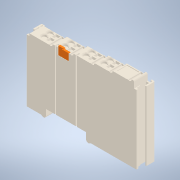
# Autodesk Inventor part: 750-530
Saved by Autodesk Inventor 2021 (Build 250183000, 183)
## iProperties
Created: 2026-07-30
Part Number: 750-530
Material: Generic
Catalog Web Link: www.3dfindit.com
Description: 750-530-8-channel digital output module 24 VDC 0.5 A high-side switching short-circuit protected
Vendor: WAGO
Document SubType Name: Modeling
Designer: psAdmin
Manufacturer: WAGO
Mass: 49.754 g
Surface Area: 192.522 cm^2
Volume: 65.9871 cm^3
Density: 1 g/cm^3
Appearance: PSOLRGB-222-214-201
Category: PARTsolutions
Company: WAGO
Title: 750-530
Author: Cadenas PARTsolutions
Comments: 8-channel digital output module 24 VDC 0.5 A high-side switching short-circuit protected
PSOL_IDENT_0: {$CADENAS_DATA/23d-libs/wago/pg15/serie750/0750-0530_0999-0962.prj},157 {VTYP=3D},{NB=750-530},{LINA=
PSOL_IDENT_1: 750-530},{NN=750-530},{DATE=29.04.2026 11:59:10},{GEOMDATE=22.04.2022 08:42:40},{VERSION=},{LINEID=1
PSOL_IDENT_2: 710},{WBVAR=},{WBNUMERIC=}  {NB=750-530},{LINA=750-530},{KT=DUMMY},{BESTNR=750-530},{INFODE=Info DE}
PSOL_IDENT_3: ,{INFOEN=Info EN},{QUERSCHNITT1=0.08 - 2.5},{QUERSCHNITT2=28 - 14},{ABISOLIERLAENGE=8 - 9},{HOEHE=64
PSOL_IDENT_4: .00},{BREITE=12.00},{TIEFE=100.00},{FARBE=lichtgrau},{GEWICHT=49.754},{BEMERKUNGEN=24V DC 0,5 A},{RG
PSOL_IDENT_5: B=0.87,0.84,0.79,0},{ECLASS71=27-24-26-04},{LINKDE=http://www.wago.com/de/p/750-530},{LINKEN=http://
PSOL_IDENT_6: www.wago.com/global/p/750-530},{FILENAME=750-530}
NB: 750-530
NN: 750-530
NT: 8-channel digital output module 24 VDC 0.5 A high-side switching short-circuit protected
NBSYN: $BESTNR.
LINA: 750-530
CATALOG: WAGO
OFFICIAL_STANDARD_NUMBERS: NO
BESTNR: 750-530
INFODE: Info DE
INFOEN: Info EN
QUERSCHNITT1: 0.08 - 2.5
QUERSCHNITT2: 28 - 14
ABISOLIERLAENGE: 8 - 9
HOEHE: 64
BREITE: 12
TIEFE: 100
FARBE: lichtgrau
GEWICHT: 49.754
BEMERKUNGEN: 24V DC 0,5 A
ECLASS71: 27-24-26-04
SUPPLIER: WAGO
ARTICLENO: 750-530
BOMINFO: 750-530
CREATOR: CADENAS GmbH
Autodesk Inventor part; units mm, degrees
ref_plane "YZ Plane" through (0, 0, 0) normal (1, 0, 0) x (0, 1, 0)
ref_plane "XZ Plane" through (0, 0, 0) normal (0, 1, 0) x (-1, 0, 0)
ref_plane "XY Plane" through (0, 0, 0) normal (0, 0, 1) x (1, 0, 0)
sketch "Skizze_1" plane through (0, 0, 0) normal (0, 0, 1) x (1, 0, 0)
  line L0 (-32.4, 49.7072) -> (-32.4, -6.4)
  line L1 (-32.4, -6.4) -> (-21.9679, -6.4)
  line L2 (-21.9679, -6.4) -> (-20.7, -7.1321)
  arc A0 (-20.7, -7.1321) -> (-17.7, -5.4) centre (-19.7, -5.4) ccw
  line L3 (-17.7, -5.4) -> (-17.7, 0)
  line L4 (-17.7, 0) -> (17.7, 0)
  line L5 (17.7, 0) -> (17.7, -5.4)
  arc A1 (17.7, -5.4) -> (20.7, -7.1321) centre (19.7, -5.4) ccw
  line L6 (20.7, -7.1321) -> (21.9679, -6.4)
  line L7 (21.9679, -6.4) -> (60, -6.4)
  line L8 (60, -6.4) -> (60, 59.4)
  arc A2 (60, 59.4) -> (59, 60.4) centre (59, 59.4) ccw
  line L9 (59, 60.4) -> (58.8171, 60.4)
  arc A3 (58.8171, 60.4) -> (58.5293, 60.2779) centre (58.8171, 60) ccw
  line L10 (58.5293, 60.2779) -> (58.4531, 60.1989)
  arc A4 (58.4531, 60.1989) -> (58.6439, 59.6405) centre (58.6915, 59.9686) ccw
  arc A5 (59.0357, 58.9584) -> (58.6439, 59.6405) centre (58.5721, 59.1457) ccw
  line L11 (59.0357, 58.9584) -> (58.9581, 58.7664)
  line L12 (58.9581, 58.7664) -> (54.8948, 57.0416)
  line L13 (54.8948, 57.0416) -> (54.7028, 57.1192)
  arc A6 (54.4842, 57.8749) -> (54.7028, 57.1192) centre (54.8901, 57.5828) ccw
  arc A7 (54.4842, 57.8749) -> (54.2152, 58.4) centre (54.2152, 58.0685) ccw
  line L14 (54.2152, 58.4) -> (41.9117, 58.4)
  line L15 (41.9117, 58.4) -> (41.8025, 58.3537)
  line L16 (41.8025, 58.3537) -> (41.6531, 58.1989)
  arc A8 (41.6531, 58.1989) -> (41.8439, 57.6405) centre (41.8915, 57.9686) ccw
  arc A9 (42.2357, 56.9584) -> (41.8439, 57.6405) centre (41.7721, 57.1457) ccw
  line L17 (42.2357, 56.9584) -> (42.1581, 56.7664)
  line L18 (42.1581, 56.7664) -> (38.0948, 55.0416)
  line L19 (38.0948, 55.0416) -> (37.9028, 55.1192)
  arc A10 (37.6842, 55.8749) -> (37.9028, 55.1192) centre (38.0901, 55.5828) ccw
  arc A11 (37.6842, 55.8749) -> (37.4152, 56.4) centre (37.4152, 56.0685) ccw
  line L20 (37.4152, 56.4) -> (25.9117, 56.4)
  line L21 (25.9117, 56.4) -> (25.8025, 56.3537)
  line L22 (25.8025, 56.3537) -> (25.6531, 56.1989)
  arc A12 (25.6531, 56.1989) -> (25.8439, 55.6405) centre (25.8915, 55.9686) ccw
  arc A13 (26.2357, 54.9584) -> (25.8439, 55.6405) centre (25.7721, 55.1457) ccw
  line L23 (26.2357, 54.9584) -> (26.1581, 54.7664)
  line L24 (26.1581, 54.7664) -> (22.0948, 53.0416)
  line L25 (22.0948, 53.0416) -> (21.9028, 53.1192)
  arc A14 (21.6842, 53.8749) -> (21.9028, 53.1192) centre (22.0901, 53.5828) ccw
  arc A15 (21.6842, 53.8749) -> (21.4152, 54.4) centre (21.4152, 54.0685) ccw
  line L26 (21.4152, 54.4) -> (7.5117, 54.4)
  line L27 (7.5117, 54.4) -> (7.4025, 54.3537)
  line L28 (7.4025, 54.3537) -> (7.2531, 54.1989)
  arc A16 (7.2531, 54.1989) -> (7.4439, 53.6405) centre (7.4915, 53.9686) ccw
  arc A17 (7.8357, 52.9584) -> (7.4439, 53.6405) centre (7.3721, 53.1457) ccw
  line L29 (7.8357, 52.9584) -> (7.7581, 52.7664)
  line L30 (7.7581, 52.7664) -> (3.6948, 51.0416)
  line L31 (3.6948, 51.0416) -> (3.5028, 51.1192)
  arc A18 (3.2842, 51.8749) -> (3.5028, 51.1192) centre (3.6901, 51.5828) ccw
  arc A19 (3.2842, 51.8749) -> (3.0152, 52.4) centre (3.0152, 52.0685) ccw
  line L32 (3.0152, 52.4) -> (-10.8883, 52.4)
  line L33 (-10.8883, 52.4) -> (-10.9975, 52.3537)
  line L34 (-10.9975, 52.3537) -> (-11.1469, 52.1989)
  arc A20 (-11.1469, 52.1989) -> (-10.9561, 51.6405) centre (-10.9085, 51.9686) ccw
  arc A21 (-10.5643, 50.9584) -> (-10.9561, 51.6405) centre (-11.0279, 51.1457) ccw
  line L35 (-10.5643, 50.9584) -> (-10.6419, 50.7664)
  line L36 (-10.6419, 50.7664) -> (-14.7052, 49.0416)
  line L37 (-14.7052, 49.0416) -> (-14.8972, 49.1192)
  arc A22 (-15.1158, 49.8749) -> (-14.8972, 49.1192) centre (-14.7099, 49.5828) ccw
  arc A23 (-15.1158, 49.8749) -> (-15.3848, 50.4) centre (-15.3848, 50.0685) ccw
  line L38 (-15.3848, 50.4) -> (-32, 50.4)
  line L39 (-32, 50.4) -> (-32.4, 49.7072)
  constraints: 80 end point, 48 point on circle, 24 centre point
extrude "Extrusion1" add sketch "Skizze_1" along normal blind 12
sketch "Skizze_10" plane through (0, 0, 0) normal (0, 0, 1) x (1, 0, 0)
  line L0 (37.2, 56.4) -> (37.9815, 54.559)
  line L1 (37.9815, 54.559) -> (42.6932, 56.559)
  line L2 (42.6932, 56.559) -> (41.9117, 58.4)
  line L3 (41.9117, 58.4) -> (41.3423, 58.1583)
  arc A0 (41.3423, 58.1583) -> (40.8125, 56.8471) centre (41.733, 57.2378) ccw
  line L4 (40.8125, 56.8471) -> (38.9715, 56.0656)
  arc A1 (38.9715, 56.0656) -> (37.6603, 56.5954) centre (38.051, 55.6749) ccw
  line L5 (37.6603, 56.5954) -> (37.2, 56.4)
  constraints: 12 end point, 4 point on circle, 2 centre point
extrude "Extrusion2" add sketch "Skizze_10" along normal blind 0.5
sketch "Skizze_11" plane through (0, 0, 0) normal (0, 0, 1) x (1, 0, 0)
  line L0 (21.2, 54.4) -> (21.9815, 52.559)
  line L1 (21.9815, 52.559) -> (26.6932, 54.559)
  line L2 (26.6932, 54.559) -> (25.9117, 56.4)
  line L3 (25.9117, 56.4) -> (25.3423, 56.1583)
  arc A0 (25.3423, 56.1583) -> (24.8125, 54.8471) centre (25.733, 55.2378) ccw
  line L4 (24.8125, 54.8471) -> (22.9715, 54.0656)
  arc A1 (22.9715, 54.0656) -> (21.6603, 54.5954) centre (22.051, 53.6749) ccw
  line L5 (21.6603, 54.5954) -> (21.2, 54.4)
  constraints: 12 end point, 4 point on circle, 2 centre point
extrude "Extrusion3" add sketch "Skizze_11" along normal blind 0.5
sketch "Skizze_12" plane through (0, 0, 0) normal (0, 0, 1) x (1, 0, 0)
  line L0 (2.8, 52.4) -> (3.5815, 50.559)
  line L1 (3.5815, 50.559) -> (8.2932, 52.559)
  line L2 (8.2932, 52.559) -> (7.5117, 54.4)
  line L3 (7.5117, 54.4) -> (6.9423, 54.1583)
  arc A0 (6.9423, 54.1583) -> (6.4125, 52.8471) centre (7.333, 53.2378) ccw
  line L4 (6.4125, 52.8471) -> (4.5715, 52.0656)
  arc A1 (4.5715, 52.0656) -> (3.2603, 52.5954) centre (3.651, 51.6749) ccw
  line L5 (3.2603, 52.5954) -> (2.8, 52.4)
  constraints: 12 end point, 4 point on circle, 2 centre point
extrude "Extrusion4" add sketch "Skizze_12" along normal blind 0.5
sketch "Skizze_13" plane through (0, 0, 0) normal (0, 0, 1) x (1, 0, 0)
  line L0 (-15.6, 50.4) -> (-14.8185, 48.559)
  line L1 (-14.8185, 48.559) -> (-10.1068, 50.559)
  line L2 (-10.1068, 50.559) -> (-10.8883, 52.4)
  line L3 (-10.8883, 52.4) -> (-11.4577, 52.1583)
  arc A0 (-11.4577, 52.1583) -> (-11.9875, 50.8471) centre (-11.067, 51.2378) ccw
  line L4 (-11.9875, 50.8471) -> (-13.8285, 50.0656)
  arc A1 (-13.8285, 50.0656) -> (-15.1397, 50.5954) centre (-14.749, 49.6749) ccw
  line L5 (-15.1397, 50.5954) -> (-15.6, 50.4)
  constraints: 12 end point, 4 point on circle, 2 centre point
extrude "Extrusion5" add sketch "Skizze_13" along normal blind 0.5
sketch "Skizze_60" plane through (0, 0, 0) normal (0, 0, 1) x (1, 0, 0)
  line L0 (54, 58.4) -> (54.7815, 56.559)
  line L1 (54.7815, 56.559) -> (59.4932, 58.559)
  line L2 (59.4932, 58.559) -> (58.7117, 60.4)
  line L3 (58.7117, 60.4) -> (58.1423, 60.1583)
  arc A0 (58.1423, 60.1583) -> (57.6125, 58.8471) centre (58.533, 59.2378) ccw
  line L4 (57.6125, 58.8471) -> (55.7715, 58.0656)
  arc A1 (55.7715, 58.0656) -> (54.4603, 58.5954) centre (54.851, 57.6749) ccw
  line L5 (54.4603, 58.5954) -> (54, 58.4)
  constraints: 12 end point, 4 point on circle, 2 centre point
extrude "Extrusion6" add sketch "Skizze_60" along normal blind 0.5
sketch "Skizze_14" plane through (0, 0, 12) normal (0, 0, 1) x (1, 0, 0)
  line L0 (37.2, 56.4) -> (37.9815, 54.559)
  line L1 (37.9815, 54.559) -> (42.6932, 56.559)
  line L2 (42.6932, 56.559) -> (41.9117, 58.4)
  line L3 (41.9117, 58.4) -> (41.3423, 58.1583)
  arc A0 (41.3423, 58.1583) -> (40.8125, 56.8471) centre (41.733, 57.2378) ccw
  line L4 (40.8125, 56.8471) -> (38.9715, 56.0656)
  arc A1 (38.9715, 56.0656) -> (37.6603, 56.5954) centre (38.051, 55.6749) ccw
  line L5 (37.6603, 56.5954) -> (37.2, 56.4)
  constraints: 12 end point, 4 point on circle, 2 centre point
extrude "Extrusion7" add sketch "Skizze_14" against normal blind 0.5
sketch "Skizze_15" plane through (0, 0, 12) normal (0, 0, 1) x (1, 0, 0)
  line L0 (21.2, 54.4) -> (21.9815, 52.559)
  line L1 (21.9815, 52.559) -> (26.6932, 54.559)
  line L2 (26.6932, 54.559) -> (25.9117, 56.4)
  line L3 (25.9117, 56.4) -> (25.3423, 56.1583)
  arc A0 (25.3423, 56.1583) -> (24.8125, 54.8471) centre (25.733, 55.2378) ccw
  line L4 (24.8125, 54.8471) -> (22.9715, 54.0656)
  arc A1 (22.9715, 54.0656) -> (21.6603, 54.5954) centre (22.051, 53.6749) ccw
  line L5 (21.6603, 54.5954) -> (21.2, 54.4)
  constraints: 12 end point, 4 point on circle, 2 centre point
extrude "Extrusion8" add sketch "Skizze_15" against normal blind 0.5
sketch "Skizze_16" plane through (0, 0, 12) normal (0, 0, 1) x (1, 0, 0)
  line L0 (2.8, 52.4) -> (3.5815, 50.559)
  line L1 (3.5815, 50.559) -> (8.2932, 52.559)
  line L2 (8.2932, 52.559) -> (7.5117, 54.4)
  line L3 (7.5117, 54.4) -> (6.9423, 54.1583)
  arc A0 (6.9423, 54.1583) -> (6.4125, 52.8471) centre (7.333, 53.2378) ccw
  line L4 (6.4125, 52.8471) -> (4.5715, 52.0656)
  arc A1 (4.5715, 52.0656) -> (3.2603, 52.5954) centre (3.651, 51.6749) ccw
  line L5 (3.2603, 52.5954) -> (2.8, 52.4)
  constraints: 12 end point, 4 point on circle, 2 centre point
extrude "Extrusion9" add sketch "Skizze_16" against normal blind 0.5
sketch "Skizze_17" plane through (0, 0, 12) normal (0, 0, 1) x (1, 0, 0)
  line L0 (-15.6, 50.4) -> (-14.8185, 48.559)
  line L1 (-14.8185, 48.559) -> (-10.1068, 50.559)
  line L2 (-10.1068, 50.559) -> (-10.8883, 52.4)
  line L3 (-10.8883, 52.4) -> (-11.4577, 52.1583)
  arc A0 (-11.4577, 52.1583) -> (-11.9875, 50.8471) centre (-11.067, 51.2378) ccw
  line L4 (-11.9875, 50.8471) -> (-13.8285, 50.0656)
  arc A1 (-13.8285, 50.0656) -> (-15.1397, 50.5954) centre (-14.749, 49.6749) ccw
  line L5 (-15.1397, 50.5954) -> (-15.6, 50.4)
  constraints: 12 end point, 4 point on circle, 2 centre point
extrude "Extrusion10" add sketch "Skizze_17" against normal blind 0.5
sketch "Skizze_61" plane through (0, 0, 12) normal (0, 0, 1) x (1, 0, 0)
  line L0 (54, 58.4) -> (54.7815, 56.559)
  line L1 (54.7815, 56.559) -> (59.4932, 58.559)
  line L2 (59.4932, 58.559) -> (58.7117, 60.4)
  line L3 (58.7117, 60.4) -> (58.1423, 60.1583)
  arc A0 (58.1423, 60.1583) -> (57.6125, 58.8471) centre (58.533, 59.2378) ccw
  line L4 (57.6125, 58.8471) -> (55.7715, 58.0656)
  arc A1 (55.7715, 58.0656) -> (54.4603, 58.5954) centre (54.851, 57.6749) ccw
  line L5 (54.4603, 58.5954) -> (54, 58.4)
  constraints: 12 end point, 4 point on circle, 2 centre point
extrude "Extrusion11" add sketch "Skizze_61" against normal blind 0.5
sketch "Skizze_46" plane through (0, 0, 12) normal (0, 0, 1) x (1, 0, 0)
  line L0 (-7.3, 46.4) -> (2.5, 46.4)
  line L1 (2.5, 46.4) -> (2.5, 52.4)
  line L2 (2.5, 52.4) -> (-7.3, 52.4)
  line L3 (-7.3, 52.4) -> (-7.3, 46.4)
  constraints: 8 end point
extrude "Extrusion12" cut sketch "Skizze_46" against normal blind 1.9
sketch "Skizze_47" plane through (0, 0, 11.05) normal (0, 0, 1) x (1, 0, 0)
  line L0 (-7, 53.4) -> (-7, 46.6)
  arc A0 (-7, 46.6) -> (-6.8, 46.4) centre (-6.8, 46.6) ccw
  line L1 (-6.8, 46.4) -> (2, 46.4)
  arc A1 (2, 46.4) -> (2.2, 46.6) centre (2, 46.6) ccw
  line L2 (2.2, 46.6) -> (2.2, 52.2)
  arc A2 (2.2, 52.2) -> (2, 52.4) centre (2, 52.2) ccw
  line L3 (2, 52.4) -> (-3.3, 52.4)
  arc A3 (-3.3305, 52.9984) -> (-3.3, 52.4) centre (-3.3, 52.7) ccw
  line L4 (-3.3305, 52.9984) -> (-2.3246, 53.1013)
  arc A4 (-2.3246, 53.1013) -> (-2.35, 53.6) centre (-2.35, 53.35) ccw
  line L5 (-2.35, 53.6) -> (-6.8, 53.6)
  arc A5 (-6.8, 53.6) -> (-7, 53.4) centre (-6.8, 53.4) ccw
  constraints: 12 end point, 12 point on circle, 6 centre point
extrude "Extrusion13" add sketch "Skizze_47" along normal mid plane 1.6
sketch "Skizze_2" plane through (0, -6.4, 0) normal (0, 1, 0) x (1, 0, 0)
  line L0 (60, 0) -> (60, -1.7)
  arc A0 (60.5, -1.2) -> (60, -1.7) centre (60.5, -1.7) ccw
  line L1 (60.5, -1.2) -> (61.9, -1.2)
  arc A1 (62.4, -1.7) -> (61.9, -1.2) centre (61.9, -1.7) ccw
  line L2 (62.4, -1.7) -> (62.4, -4.3)
  arc A2 (62.4, -4.3) -> (63.8, -4.3) centre (63.1, -4.3) ccw
  line L3 (63.8, -4.3) -> (63.8, 1.8)
  arc A3 (63.8, 1.8) -> (62.8, 2.8) centre (62.8, 1.8) ccw
  line L4 (62.8, 2.8) -> (61.3, 2.8)
  arc A4 (61.3, 2.8) -> (60.8, 2.3) centre (61.3, 2.3) ccw
  line L5 (60.8, 2.3) -> (60.8, 1.9)
  arc A5 (60.8, 1.9) -> (61, 1.7) centre (61, 1.9) ccw
  line L6 (61, 1.7) -> (62.2, 1.7)
  arc A6 (62.4, 1.5) -> (62.2, 1.7) centre (62.2, 1.5) ccw
  line L7 (62.4, 1.5) -> (62.4, 0.2)
  arc A7 (62.2, 0) -> (62.4, 0.2) centre (62.2, 0.2) ccw
  line L8 (62.2, 0) -> (60, 0)
  constraints: 18 end point, 16 point on circle, 8 centre point
extrude "Extrusion14" add sketch "Skizze_2" along normal blind 60.8
sketch "Skizze_3" plane through (0, -6.4, 0) normal (0, 1, 0) x (1, 0, 0)
  arc A0 (-36.2, -4.3) -> (-34.8, -4.3) centre (-35.5, -4.3) ccw
  line L0 (-34.8, -4.3) -> (-34.8, -1.7)
  arc A1 (-34.3, -1.2) -> (-34.8, -1.7) centre (-34.3, -1.7) ccw
  line L1 (-34.3, -1.2) -> (-32.9, -1.2)
  arc A2 (-32.4, -1.7) -> (-32.9, -1.2) centre (-32.9, -1.7) ccw
  line L2 (-32.4, -1.7) -> (-32.4, 0)
  line L3 (-32.4, 0) -> (-34.6, 0)
  arc A3 (-34.8, 0.2) -> (-34.6, 0) centre (-34.6, 0.2) ccw
  line L4 (-34.8, 0.2) -> (-34.8, 1.5)
  arc A4 (-34.6, 1.7) -> (-34.8, 1.5) centre (-34.6, 1.5) ccw
  line L5 (-34.6, 1.7) -> (-33.4, 1.7)
  arc A5 (-33.4, 1.7) -> (-33.2, 1.9) centre (-33.4, 1.9) ccw
  line L6 (-33.2, 1.9) -> (-33.2, 2.3)
  arc A6 (-33.2, 2.3) -> (-33.7, 2.8) centre (-33.7, 2.3) ccw
  line L7 (-33.7, 2.8) -> (-35.2, 2.8)
  arc A7 (-35.2, 2.8) -> (-36.2, 1.8) centre (-35.2, 1.8) ccw
  line L8 (-36.2, 1.8) -> (-36.2, -4.3)
  constraints: 18 end point, 16 point on circle, 8 centre point
extrude "Extrusion15" add sketch "Skizze_3" along normal blind 54.8
sketch "Skizze_9" plane through (0, -6.4, 0) normal (0, 1, 0) x (1, 0, 0)
  line L0 (-34.6, -10.6) -> (-34.6, -11.8)
  arc A0 (-34.6, -11.8) -> (-34.4, -12) centre (-34.4, -11.8) ccw
  line L1 (-34.4, -12) -> (-32.4, -12)
  line L2 (-32.4, -12) -> (-32.4, -7)
  line L3 (-32.4, -7) -> (-33, -7)
  line L4 (-33, -7) -> (-33, -10.4)
  line L5 (-33, -10.4) -> (-34.4, -10.4)
  arc A1 (-34.4, -10.4) -> (-34.6, -10.6) centre (-34.4, -10.6) ccw
  constraints: 12 end point, 4 point on circle, 2 centre point
extrude "Extrusion16" add sketch "Skizze_9" along normal blind 54.8
sketch "Skizze_8" plane through (0, -6.4, 0) normal (0, 1, 0) x (1, 0, 0)
  line L0 (60, -7) -> (60, -12)
  line L1 (60, -12) -> (62, -12)
  arc A0 (62, -12) -> (62.2, -11.8) centre (62, -11.8) ccw
  line L2 (62.2, -11.8) -> (62.2, -10.6)
  arc A1 (62.2, -10.6) -> (62, -10.4) centre (62, -10.6) ccw
  line L3 (62, -10.4) -> (60.6, -10.4)
  line L4 (60.6, -10.4) -> (60.6, -7)
  line L5 (60.6, -7) -> (60, -7)
  constraints: 12 end point, 4 point on circle, 2 centre point
extrude "Extrusion17" add sketch "Skizze_8" along normal blind 60.8
sketch "Sketch18" plane through (25.9117, 56.4, 12) normal (0, 1, 0) x (1, 0, 0)
  point P0 (3.1883, 9.5)
hole "Hole1" at (29.1, 56.4, 2.5) direction (0, -1, 0) diameter 4.2 depth 2 countersink diameter 5.4 countersink angle 90
pattern_linear "Rectangular Pattern1" count 2 spacing 5 along (0, 0, 1) of "Hole1"
sketch "Skizze_24" plane through (31.2, 0, 0) normal (1, 0, 0) x (0, 0, -1)
  line L0 (-2.5, 54.4) -> (-2.5, 56.4)
  line L1 (-2.5, 56.4) -> (-1.2, 56.4)
  line L2 (-1.2, 56.4) -> (-1.4, 55.8)
  line L3 (-1.4, 55.8) -> (-1.4, 54.4)
  line L4 (-1.4, 54.4) -> (-2.5, 54.4)
  line L5 (-2.5, 54.4) -> (-2.5, 56.4)
  constraints: 12 end point
revolve "Revolution1" cut sketch "Skizze_24" angle 360 about axis through (31.2, 54.4, 2.5) along (0, -1, 0)
pattern_linear "Rectangular Pattern2" count 2 spacing 5 along (0, 0, 1) of "Revolution1"
sketch "Skizze_26" plane through (33, 0, 0) normal (1, 0, 0) x (0, 0, -1)
  line L0 (-4.5, 54.4) -> (-0.8, 54.4)
  line L1 (-0.8, 54.4) -> (-0.8, 56.4)
  line L2 (-0.8, 56.4) -> (-4.5, 56.4)
  line L3 (-4.5, 56.4) -> (-4.5, 54.4)
  constraints: 8 end point
extrude "Extrusion18" cut sketch "Skizze_26" along normal blind 3.8
pattern_linear "Rectangular Pattern3" count 2 spacing 5 along (0, 0, 1) of "Extrusion18"
sketch "Sketch21" plane through (7.5117, 54.4, 12) normal (0, 1, 0) x (1, 0, 0)
  point P0 (5.5883, 9.5)
hole "Hole2" at (13.1, 54.4, 2.5) direction (0, -1, 0) diameter 4.2 depth 2 countersink diameter 5.4 countersink angle 90
pattern_linear "Rectangular Pattern4" count 2 spacing 5 along (0, 0, 1) of "Hole2"
sketch "Skizze_30" plane through (15.2, 0, 0) normal (1, 0, 0) x (0, 0, -1)
  line L0 (-2.5, 52.4) -> (-2.5, 54.4)
  line L1 (-2.5, 54.4) -> (-1.2, 54.4)
  line L2 (-1.2, 54.4) -> (-1.4, 53.8)
  line L3 (-1.4, 53.8) -> (-1.4, 52.4)
  line L4 (-1.4, 52.4) -> (-2.5, 52.4)
  line L5 (-2.5, 52.4) -> (-2.5, 54.4)
  constraints: 12 end point
revolve "Revolution2" cut sketch "Skizze_30" angle 360 about axis through (15.2, 52.4, 2.5) along (0, -1, 0)
pattern_linear "Rectangular Pattern5" count 2 spacing 5 along (0, 0, 1) of "Revolution2"
sketch "Skizze_32" plane through (17, 0, 0) normal (1, 0, 0) x (0, 0, -1)
  line L0 (-4.5, 52.4) -> (-0.8, 52.4)
  line L1 (-0.8, 52.4) -> (-0.8, 54.4)
  line L2 (-0.8, 54.4) -> (-4.5, 54.4)
  line L3 (-4.5, 54.4) -> (-4.5, 52.4)
  constraints: 8 end point
extrude "Extrusion19" cut sketch "Skizze_32" along normal blind 3.8
pattern_linear "Rectangular Pattern6" count 2 spacing 5 along (0, 0, 1) of "Extrusion19"
sketch "Sketch24" plane through (-10.8883, 52.4, 12) normal (0, 1, 0) x (1, 0, 0)
  point P0 (5.5883, 9.5)
hole "Hole3" at (-5.3, 52.4, 2.5) direction (0, -1, 0) diameter 4.2 depth 2 countersink diameter 5.4 countersink angle 90
pattern_linear "Rectangular Pattern7" count 2 spacing 5 along (0, 0, 1) of "Hole3"
sketch "Skizze_36" plane through (-3.2, 0, 0) normal (1, 0, 0) x (0, 0, -1)
  line L0 (-2.5, 50.4) -> (-2.5, 52.4)
  line L1 (-2.5, 52.4) -> (-1.2, 52.4)
  line L2 (-1.2, 52.4) -> (-1.4, 51.8)
  line L3 (-1.4, 51.8) -> (-1.4, 50.4)
  line L4 (-1.4, 50.4) -> (-2.5, 50.4)
  line L5 (-2.5, 50.4) -> (-2.5, 52.4)
  constraints: 12 end point
revolve "Revolution3" cut sketch "Skizze_36" angle 360 about axis through (-3.2, 50.4, 2.5) along (0, -1, 0)
pattern_linear "Rectangular Pattern8" count 2 spacing 5 along (0, 0, 1) of "Revolution3"
sketch "Skizze_38" plane through (-1.4, 0, 0) normal (1, 0, 0) x (0, 0, -1)
  line L0 (-4.5, 50.4) -> (-0.8, 50.4)
  line L1 (-0.8, 50.4) -> (-0.8, 52.4)
  line L2 (-0.8, 52.4) -> (-4.5, 52.4)
  line L3 (-4.5, 52.4) -> (-4.5, 50.4)
  constraints: 8 end point
extrude "Extrusion20" cut sketch "Skizze_38" along normal blind 3.8
pattern_linear "Rectangular Pattern9" count 2 spacing 5 along (0, 0, 1) of "Extrusion20"
sketch "Sketch27" plane through (-32, 50.4, 12) normal (0, 1, 0) x (1, 0, 0)
  point P0 (8.3, 9.5)
hole "Hole4" at (-23.7, 50.4, 2.5) direction (0, -1, 0) diameter 4.2 depth 2 countersink diameter 5.4 countersink angle 90
pattern_linear "Rectangular Pattern10" count 2 spacing 5 along (0, 0, 1) of "Hole4"
sketch "Skizze_42" plane through (-21.6, 0, 0) normal (1, 0, 0) x (0, 0, -1)
  line L0 (-2.5, 48.4) -> (-2.5, 50.4)
  line L1 (-2.5, 50.4) -> (-1.2, 50.4)
  line L2 (-1.2, 50.4) -> (-1.4, 49.8)
  line L3 (-1.4, 49.8) -> (-1.4, 48.4)
  line L4 (-1.4, 48.4) -> (-2.5, 48.4)
  line L5 (-2.5, 48.4) -> (-2.5, 50.4)
  constraints: 12 end point
revolve "Revolution4" cut sketch "Skizze_42" angle 360 about axis through (-21.6, 48.4, 2.5) along (0, -1, 0)
pattern_linear "Rectangular Pattern11" count 2 spacing 5 along (0, 0, 1) of "Revolution4"
sketch "Skizze_44" plane through (-19.8, 0, 0) normal (1, 0, 0) x (0, 0, -1)
  line L0 (-4.5, 48.4) -> (-0.8, 48.4)
  line L1 (-0.8, 48.4) -> (-0.8, 50.4)
  line L2 (-0.8, 50.4) -> (-4.5, 50.4)
  line L3 (-4.5, 50.4) -> (-4.5, 48.4)
  constraints: 8 end point
extrude "Extrusion21" cut sketch "Skizze_44" along normal blind 3.8
pattern_linear "Rectangular Pattern12" count 2 spacing 5 along (0, 0, 1) of "Extrusion21"
sketch "Skizze_4" plane through (0, 0, 1) normal (0, 0, 1) x (1, 0, 0)
  line L0 (42.9, 57.9) -> (53.7, 57.9)
  line L1 (53.7, 57.9) -> (53.7, 58.4)
  line L2 (53.7, 58.4) -> (42.9, 58.4)
  line L3 (42.9, 58.4) -> (42.9, 57.9)
  constraints: 8 end point
extrude "Extrusion22" cut sketch "Skizze_4" along normal blind 9.05
sketch "Sketch_1" plane through (0, 0, 0) normal (0, 1, 0) x (-1, 0, 0)
  line L0 (9.7, 13) -> (-9.7, 13)
  line L1 (-9.7, 13) -> (-9.7, 9.4)
  line L2 (-9.7, 9.4) -> (-8.7, 9.4)
  line L3 (-8.7, 9.4) -> (-8.7, 12)
  line L4 (-8.7, 12) -> (8.7, 12)
  line L5 (8.7, 12) -> (8.7, 9.4)
  line L6 (8.7, 9.4) -> (9.7, 9.4)
  line L7 (9.7, 9.4) -> (9.7, 13)
  constraints: 16 end point
extrude "Extrusion23" cut sketch "Sketch_1" along normal blind 55
sketch "Sketch_2" plane through (0, 0, 0) normal (0, 0, 1) x (1, 0, 0)
  line L0 (8.95, 44.9) -> (8.95, 41.3)
  line L1 (8.95, 41.3) -> (9.35, 41.3)
  line L2 (9.35, 41.3) -> (9.35, 44.9)
  line L3 (9.35, 44.9) -> (8.95, 44.9)
  constraints: 8 end point
extrude "Extrusion24" add sketch "Sketch_2" against normal blind 2.4
sketch "Sketch_3" plane through (0, 0, 0) normal (0, 0, 1) x (1, 0, 0)
  line L0 (-9.45, 42.9) -> (-9.45, 39.3)
  line L1 (-9.45, 39.3) -> (-9.05, 39.3)
  line L2 (-9.05, 39.3) -> (-9.05, 42.9)
  line L3 (-9.05, 42.9) -> (-9.45, 42.9)
  constraints: 8 end point
extrude "Extrusion25" add sketch "Sketch_3" against normal blind 2.4
ref_plane "1_10_XY" through (-17.9, 50.4, 2.65) normal (0, 1, 0) x (1, 0, 0)
ref_plane "1_10_YZ" through (-17.9, 50.4, 2.65) normal (1, 0, 0) x (0, 0, -1)
ref_plane "1_10_ZX" through (-17.9, 50.4, 2.65) normal (0, 0, -1) x (0, 1, 0)
ref_plane "1_11_XY" through (-17.9, 50.4, 7.65) normal (0, 1, 0) x (1, 0, 0)
ref_plane "1_11_YZ" through (-17.9, 50.4, 7.65) normal (1, 0, 0) x (0, 0, -1)
ref_plane "1_11_ZX" through (-17.9, 50.4, 7.65) normal (0, 0, -1) x (0, 1, 0)
ref_plane "1_12_XY" through (0.5, 52.4, 2.65) normal (0, 1, 0) x (1, 0, 0)
ref_plane "1_12_YZ" through (0.5, 52.4, 2.65) normal (1, 0, 0) x (0, 0, -1)
ref_plane "1_12_ZX" through (0.5, 52.4, 2.65) normal (0, 0, -1) x (0, 1, 0)
ref_plane "1_13_XY" through (0.5, 52.4, 7.65) normal (0, 1, 0) x (1, 0, 0)
ref_plane "1_13_YZ" through (0.5, 52.4, 7.65) normal (1, 0, 0) x (0, 0, -1)
ref_plane "1_13_ZX" through (0.5, 52.4, 7.65) normal (0, 0, -1) x (0, 1, 0)
ref_plane "1_14_XY" through (18.9, 54.4, 2.65) normal (0, 1, 0) x (1, 0, 0)
ref_plane "1_14_YZ" through (18.9, 54.4, 2.65) normal (1, 0, 0) x (0, 0, -1)
ref_plane "1_14_ZX" through (18.9, 54.4, 2.65) normal (0, 0, -1) x (0, 1, 0)
ref_plane "1_15_XY" through (18.9, 54.4, 7.65) normal (0, 1, 0) x (1, 0, 0)
ref_plane "1_15_YZ" through (18.9, 54.4, 7.65) normal (1, 0, 0) x (0, 0, -1)
ref_plane "1_15_ZX" through (18.9, 54.4, 7.65) normal (0, 0, -1) x (0, 1, 0)
ref_plane "1_16_XY" through (34.9, 56.4, 2.65) normal (0, 1, 0) x (1, 0, 0)
ref_plane "1_16_YZ" through (34.9, 56.4, 2.65) normal (1, 0, 0) x (0, 0, -1)
ref_plane "1_16_ZX" through (34.9, 56.4, 2.65) normal (0, 0, -1) x (0, 1, 0)
ref_plane "1_17_XY" through (34.9, 56.4, 7.65) normal (0, 1, 0) x (1, 0, 0)
ref_plane "1_17_YZ" through (34.9, 56.4, 7.65) normal (1, 0, 0) x (0, 0, -1)
ref_plane "1_17_ZX" through (34.9, 56.4, 7.65) normal (0, 0, -1) x (0, 1, 0)
ref_plane "1_18_XY" through (-12.6736, 49.904, 2.5) normal (-0.3907311, 0.9205049, 0) x (0.9205049, 0.3907311, 0)
ref_plane "1_18_YZ" through (-12.6736, 49.904, 2.5) normal (0.9205049, 0.3907311, 0) x (0, 0, -1)
ref_plane "1_18_ZX" through (-12.6736, 49.904, 2.5) normal (0, 0, -1) x (-0.3907311, 0.9205049, 0)
ref_plane "1_19_XY" through (-12.6736, 49.904, 7.5) normal (-0.3907311, 0.9205049, 0) x (0.9205049, 0.3907311, 0)
ref_plane "1_19_YZ" through (-12.6736, 49.904, 7.5) normal (0.9205049, 0.3907311, 0) x (0, 0, -1)
ref_plane "1_19_ZX" through (-12.6736, 49.904, 7.5) normal (0, 0, -1) x (-0.3907311, 0.9205049, 0)
ref_plane "1_2_XY" through (-23.7, 50.4, 2.5) normal (0, 1, 0) x (1, 0, 0)
ref_plane "1_2_YZ" through (-23.7, 50.4, 2.5) normal (1, 0, 0) x (0, 0, -1)
ref_plane "1_2_ZX" through (-23.7, 50.4, 2.5) normal (0, 0, -1) x (0, 1, 0)
ref_plane "1_20_XY" through (5.7264, 51.904, 2.5) normal (-0.3907311, 0.9205049, 0) x (0.9205049, 0.3907311, 0)
ref_plane "1_20_YZ" through (5.7264, 51.904, 2.5) normal (0.9205049, 0.3907311, 0) x (0, 0, -1)
ref_plane "1_20_ZX" through (5.7264, 51.904, 2.5) normal (0, 0, -1) x (-0.3907311, 0.9205049, 0)
ref_plane "1_21_XY" through (5.7264, 51.904, 7.5) normal (-0.3907311, 0.9205049, 0) x (0.9205049, 0.3907311, 0)
ref_plane "1_21_YZ" through (5.7264, 51.904, 7.5) normal (0.9205049, 0.3907311, 0) x (0, 0, -1)
ref_plane "1_21_ZX" through (5.7264, 51.904, 7.5) normal (0, 0, -1) x (-0.3907311, 0.9205049, 0)
ref_plane "1_22_XY" through (24.1264, 53.904, 2.5) normal (-0.3907311, 0.9205049, 0) x (0.9205049, 0.3907311, 0)
ref_plane "1_22_YZ" through (24.1264, 53.904, 2.5) normal (0.9205049, 0.3907311, 0) x (0, 0, -1)
ref_plane "1_22_ZX" through (24.1264, 53.904, 2.5) normal (0, 0, -1) x (-0.3907311, 0.9205049, 0)
ref_plane "1_23_XY" through (24.1264, 53.904, 7.5) normal (-0.3907311, 0.9205049, 0) x (0.9205049, 0.3907311, 0)
ref_plane "1_23_YZ" through (24.1264, 53.904, 7.5) normal (0.9205049, 0.3907311, 0) x (0, 0, -1)
ref_plane "1_23_ZX" through (24.1264, 53.904, 7.5) normal (0, 0, -1) x (-0.3907311, 0.9205049, 0)
ref_plane "1_24_XY" through (40.1264, 55.904, 2.5) normal (-0.3907311, 0.9205049, 0) x (0.9205049, 0.3907311, 0)
ref_plane "1_24_YZ" through (40.1264, 55.904, 2.5) normal (0.9205049, 0.3907311, 0) x (0, 0, -1)
ref_plane "1_24_ZX" through (40.1264, 55.904, 2.5) normal (0, 0, -1) x (-0.3907311, 0.9205049, 0)
ref_plane "1_25_XY" through (40.1264, 55.904, 7.5) normal (-0.3907311, 0.9205049, 0) x (0.9205049, 0.3907311, 0)
ref_plane "1_25_YZ" through (40.1264, 55.904, 7.5) normal (0.9205049, 0.3907311, 0) x (0, 0, -1)
ref_plane "1_25_ZX" through (40.1264, 55.904, 7.5) normal (0, 0, -1) x (-0.3907311, 0.9205049, 0)
ref_plane "1_27_XY" through (56.9264, 57.904, 2.5) normal (-0.3907311, 0.9205049, 0) x (0.9205049, 0.3907311, 0)
ref_plane "1_27_YZ" through (56.9264, 57.904, 2.5) normal (0.9205049, 0.3907311, 0) x (0, 0, -1)
ref_plane "1_27_ZX" through (56.9264, 57.904, 2.5) normal (0, 0, -1) x (-0.3907311, 0.9205049, 0)
ref_plane "1_28_XY" through (56.9264, 57.904, 7.5) normal (-0.3907311, 0.9205049, 0) x (0.9205049, 0.3907311, 0)
ref_plane "1_28_YZ" through (56.9264, 57.904, 7.5) normal (0.9205049, 0.3907311, 0) x (0, 0, -1)
ref_plane "1_28_ZX" through (56.9264, 57.904, 7.5) normal (0, 0, -1) x (-0.3907311, 0.9205049, 0)
ref_plane "1_3_XY" through (-23.7, 50.4, 7.5) normal (0, 1, 0) x (1, 0, 0)
ref_plane "1_3_YZ" through (-23.7, 50.4, 7.5) normal (1, 0, 0) x (0, 0, -1)
ref_plane "1_3_ZX" through (-23.7, 50.4, 7.5) normal (0, 0, -1) x (0, 1, 0)
ref_plane "1_4_XY" through (-5.3, 52.4, 2.5) normal (0, 1, 0) x (1, 0, 0)
ref_plane "1_4_YZ" through (-5.3, 52.4, 2.5) normal (1, 0, 0) x (0, 0, -1)
ref_plane "1_4_ZX" through (-5.3, 52.4, 2.5) normal (0, 0, -1) x (0, 1, 0)
ref_plane "1_5_XY" through (-5.3, 52.4, 7.5) normal (0, 1, 0) x (1, 0, 0)
ref_plane "1_5_YZ" through (-5.3, 52.4, 7.5) normal (1, 0, 0) x (0, 0, -1)
ref_plane "1_5_ZX" through (-5.3, 52.4, 7.5) normal (0, 0, -1) x (0, 1, 0)
ref_plane "1_6_XY" through (13.1, 54.4, 2.5) normal (0, 1, 0) x (1, 0, 0)
ref_plane "1_6_YZ" through (13.1, 54.4, 2.5) normal (1, 0, 0) x (0, 0, -1)
ref_plane "1_6_ZX" through (13.1, 54.4, 2.5) normal (0, 0, -1) x (0, 1, 0)
ref_plane "1_7_XY" through (13.1, 54.4, 7.5) normal (0, 1, 0) x (1, 0, 0)
ref_plane "1_7_YZ" through (13.1, 54.4, 7.5) normal (1, 0, 0) x (0, 0, -1)
ref_plane "1_7_ZX" through (13.1, 54.4, 7.5) normal (0, 0, -1) x (0, 1, 0)
ref_plane "1_8_XY" through (29.1, 56.4, 2.5) normal (0, 1, 0) x (1, 0, 0)
ref_plane "1_8_YZ" through (29.1, 56.4, 2.5) normal (1, 0, 0) x (0, 0, -1)
ref_plane "1_8_ZX" through (29.1, 56.4, 2.5) normal (0, 0, -1) x (0, 1, 0)
ref_plane "1_9_XY" through (29.1, 56.4, 7.5) normal (0, 1, 0) x (1, 0, 0)
ref_plane "1_9_YZ" through (29.1, 56.4, 7.5) normal (1, 0, 0) x (0, 0, -1)
ref_plane "1_9_ZX" through (29.1, 56.4, 7.5) normal (0, 0, -1) x (0, 1, 0)
body "Solid1"
